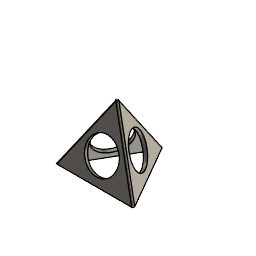
day15-painters-tripod (Autodesk Fusion 360 design; units mm, degrees)
part number: 2026-06-13-23-10-56-739
Autodesk Fusion 360 part; units mm, degrees
sketch "Bottom Contour" plane through (0, 0, 0) normal (0, 0, 1) x (1, 0, 0)
  line L0 (0, 0) -> (30, 51.9615)
  line L1 (30, 51.9615) -> (60, 0)
  line L2 (60, 0) -> (0, 0)
  dimension "d1" = 60
  constraint coincident L0.start L2.end
  constraint horizontal L2
  constraint equal L0 L1
  constraint equal L1 L2
  measures "d1" distance of L0.start L0.end
ref_plane "WorkPlane1" through (0, 0, 50) normal (0, 0, 1) x (1, 0, 0)
sketch "Top Point" plane through (0, 0, 50) normal (0, 0, 1) x (1, 0, 0)
  line L0 (0, 0) -> (30, 51.9615)
  line L1 (30, 51.9615) -> (60, 0)
  line L2 (60, 0) -> (0, 0)
  line L3 (30, 51.9615) -> (30, 0) construction
  line L4 (45, 25.9808) -> (0, 0) construction
  point P0 (30, 17.3205)
  constraint coincident L0.end L1.start
  constraint midpoint L2 L3.end
  constraint midpoint L1 L4.start
  constraint coincident L0.start L2.end
  constraint coincident L3 P0
  constraint coincident L4 P0
loft "Loft1" add profiles "Bottom Contour" section 1 section 2 point at (30, 17.3205, 50)
shell "Shell1" thickness 2.5 removed faces 1 at (30, 17.3205, 0)
sketch "Sketch3" plane through (0, 0, 0) normal (0, -0.944911, 0.327327) x (1, 0, 0)
  line L0 (0, 0) -> (60, 0)
  line L1 (60, 0) -> (30, 52.915)
  line L2 (30, 52.915) -> (0, 0)
  line L3 (30, 52.915) -> (30, 0) construction
  line L4 (45, 26.4575) -> (0, 0) construction
  circle A0 centre (30, 17.6383) radius 12.5
  dimension "d4" = 25
  constraint coincident L1.end L2.start
  constraint midpoint L0 L3.end
  constraint midpoint L1 L4.start
  constraint coincident L0.start L2.end
  constraint coincident L3 A0.centre
  constraint coincident L4 A0.centre
  measures "d4" diameter of A0
extrude "Extrude1" cut sketch "Sketch3" against normal up to surface (2.5 mm away) contours A0
pattern_circular "C-Pattern1" count 3 over 360 about axis through (30, 17.3205, 75) along (0, 0, -1) of "Extrude1"
fillet "Fillet1" radius 1 3 edges at (15, 8.6603, 25) (45, 8.6603, 25) (30, 34.641, 25)
